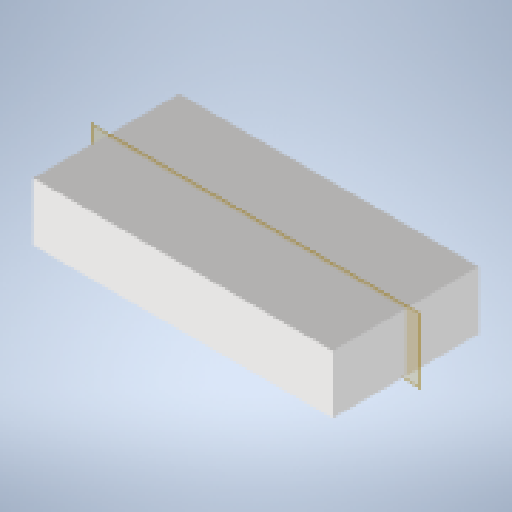
# Autodesk Inventor part: LinearRailBlock
Saved by Autodesk Inventor 2023 (Build 270158000, 158)
## iProperties
Created: 2023-09-03
Part Number: LinearRailBlock
Material: Steel, Carbon
Document SubType Name: Modeling
Designer: Felix
Density: 7.85 g/cm^3
Appearance: Semi-Polished
Author: Felix
Autodesk Inventor part; units mm, degrees
ref_plane "YZ Plane" through (0, 0, 0) normal (1, 0, 0) x (0, 1, 0)
ref_plane "XZ Plane" through (0, 0, 0) normal (0, 1, 0) x (-1, 0, 0)
ref_plane "XY Plane" through (0, 0, 0) normal (0, 0, 1) x (1, 0, 0)
sketch "Sketch1" plane through (0, 0, 0) normal (0, 1, 0) x (-1, 0, 0)
  line L0 (-20.5, 10) -> (20.5, 10)
  line L1 (20.5, 10) -> (20.5, -10)
  line L2 (20.5, -10) -> (-20.5, -10)
  line L3 (-20.5, -10) -> (-20.5, 10)
  line L4 (-20.5, 10) -> (20.5, -10) construction
  line L5 (20.5, 10) -> (-20.5, -10) construction
  point P0 (0, 0)
  dimension "d0" = 41
  dimension "d1" = 20
  constraints: 12 end point, 2 midpoint, 2 parallel, 1 horizontal, 1 perpendicular
  measures "d0" distance of L1.end L2.end
  measures "d1" distance of L0.end L1.end
extrude "Extrusion1" add sketch "Sketch1" along normal blind 8
ref_plane "Work Plane1" through (20.5, 0, 0) normal (0, 0, 1) x (1, 0, 0)
sketch "Sketch2" plane through (0, 0, 0) normal (0, -1, 0) x (1, 0, 0)
  line L0 (20.5, -10) -> (-20.5, -10) construction
  line L1 (20.5, 10) -> (20.5, -10) construction
  line L2 (-20.5, 10) -> (20.5, 10) construction
  line L3 (-20.5, -10) -> (-20.5, 10) construction
  line L4 (-8, -7.5) -> (8, -7.5) construction
  line L5 (8, -7.5) -> (8, 7.5) construction
  line L6 (8, 7.5) -> (-8, 7.5) construction
  line L7 (-8, 7.5) -> (-8, -7.5) construction
  line L8 (-8, -7.5) -> (8, 7.5) construction
  line L9 (8, -7.5) -> (-8, 7.5) construction
  point P0 (0, 0)
  dimension "d4" = 16
  dimension "d5" = 15
  constraints: 12 end point, 2 midpoint, 2 parallel, 1 horizontal, 1 perpendicular
  measures "d4" distance of L6.end L5.end
  measures "d5" distance of L4.end L5.end
hole "Hole1" at (8, 0, -7.5) at (8, 0, 7.5) at (-8, 0, 7.5) at (-8, 0, -7.5) direction (0, 1, 0) diameter 2.459 depth 4 thread size "M3x0.5" class "6H" standard "ISO Metric profile"
body "Solid1"
